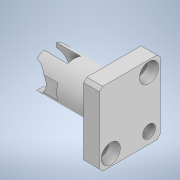
# Autodesk Inventor part: Фиксатор-11
Saved by Autodesk Inventor 2022 (Build 260153000, 153)
## iProperties
Created: 2021-12-02
Part Number: Фиксатор-11
Material: Типовые
Document SubType Name: Modeling
Designer: Украинцев
Density: 1 g/cm^3
Appearance: По умолчанию
Author: Украинцев
Autodesk Inventor part; units mm, degrees
ref_plane "YZ Plane" through (0, 0, 0) normal (1, 0, 0) x (0, 1, 0)
ref_plane "XZ Plane" through (0, 0, 0) normal (0, 1, 0) x (-1, 0, 0)
ref_plane "XY Plane" through (0, 0, 0) normal (0, 0, 1) x (1, 0, 0)
sketch "Эскиз1" plane through (0, 0, 0) normal (0, 1, 0) x (-1, 0, 0)
  line L0 (-5, -19) -> (5, -19)
  line L1 (5, -19) -> (5, 19)
  line L2 (5, 19) -> (-5, 19)
  line L3 (-5, 19) -> (-5, -19)
  line L4 (-5, -19) -> (5, 19) construction
  line L5 (5, -19) -> (-5, 19) construction
  line L6 (5, 0) -> (5, 12)
  line L7 (5, 12) -> (45, 12)
  line L8 (45, 12) -> (45, 0)
  line L9 (30, 0) -> (5, 0)
  line L10 (45, 0) -> (45, 4)
  line L11 (45, 4) -> (30, 4)
  line L12 (30, 4) -> (30, 0)
  line L13 (45, 12) -> (45, 11)
  line L14 (45, 11) -> (29, 11)
  line L15 (29, 11) -> (29, 12)
  line L16 (45, 4) -> (30, 4)
  line L17 (30, 4) -> (30, -4)
  line L18 (30, -4) -> (45, -4)
  line L19 (45, -4) -> (45, 4)
  line L20 (29, -11) -> (29, -12)
  line L21 (29, -12) -> (45, -12)
  line L22 (45, -12) -> (45, -11)
  line L23 (45, -11) -> (29, -11)
  line L24 (29, -11) -> (29, -12)
  line L25 (5, 12) -> (8, 12)
  line L26 (5, 0) -> (5, 11.75)
  line L27 (5, 11.75) -> (8, 11.75)
  line L28 (8, 11.75) -> (8, 12)
  line L29 (5, 11.75) -> (6, 11.75)
  line L30 (6, 11.75) -> (6, 12.75)
  line L31 (6, 12.75) -> (5, 12.75)
  line L32 (5, 12.75) -> (5, 11.75)
  circle A0 centre (6, 12.75) radius 1
  line L33 (8, 12) -> (6, 11.75)
  point P0 (0, 0)
  point P1 (6.2462, 11.7808)
  dimension "d0" = 10
  dimension "d1" = 38
  dimension "d2" = 12
  dimension "d3" = 40
  dimension "d4" = 4
  dimension "d5" = 15
  dimension "d6" = 1
  dimension "d7" = 16
  dimension "d13" = 8
  dimension "d14" = 22
  dimension "d15" = 1
  dimension "d60" = 3
  dimension "d61" = 11.75
  dimension "d62" = 1
  dimension "d63" = 1
  constraints: 68 end point, 12 perpendicular, 8 parallel, 6 point on line, 5 horizontal, 4 midpoint, 1 centre point, 1 coincident, 1 tangent
  measures "d0" distance of L2.end L1.end
  measures "d1" distance of L1.end L0.end
  measures "d2" distance of L6.start L6.end
  measures "d3" distance of L6.end L7.end
  measures "d4" distance of L8.end L10.end
  measures "d5" distance of L10.end L11.end
  measures "d6" distance of L7.end L13.end
  measures "d7" distance of L13.end L14.end
  measures "d13" distance of L17.end L16.end
  measures "d14" distance of L14.end L20.start
  measures "d15" distance of L20.start L20.end
  measures "d60" distance of L6.end L25.end
  measures "d61" distance of L6.start L26.end
  measures "d62" distance of L31.end L30.end
  measures "d63" distance of L30.end L29.end
extrude "Выдавливание1" add sketch "Эскиз1" along normal mid plane 46 contours L3 L2 L1 L0
revolve "Вращение1" add sketch "Эскиз1" angle 360 about axis through (-30, 0, 0) along (1, 0, 0) contours L1 L27 L28 L7 L15 L14 L8 L11 L12 L9 | L1 L7 A0 L27 | A0 L7 L1 | A0 L33 L28 L27 | L14 L15 L7 L8
extrude "Выдавливание3" cut sketch "Эскиз1" along normal mid plane 46 contours L12 L11 L8 L19 L18 L17 | L14 L15 L7 L8 | L23 L22 L21 L20
sketch "Эскиз3" plane through (-29, 4.7958, -11) normal (0, 0, -1) x (-1, 0, 0)
  line L0 (16, -9.5917) -> (16, 0) projected
  circle A0 centre (16, -4.7958) radius 8.5
  point P0 (-29, -4.7958)
  dimension "d21" = 17
  constraints: 1 centre point, 1 midpoint
  measures "d21" diameter of A0
extrude "Выдавливание5" cut sketch "Эскиз3" against normal blind 39
sketch "Эскиз4" plane through (5, -23, -19) normal (1, 0, 0) x (0, 0, -1)
  line L0 (-19, 23) -> (-19, 39)
  line L1 (-19, 39) -> (-31, 39)
  line L2 (-19, 23) -> (-19, 7)
  line L3 (-19, 7) -> (-7, 7)
  line L4 (-19, 7) -> (-31, 7)
  line L5 (-19, 39) -> (-7, 39)
  dimension "d24" = 16
  dimension "d25" = 12
  dimension "d26" = 16
  dimension "d27" = 12
  dimension "d28" = 12
  constraints: 12 end point, 4 coincident, 3 perpendicular, 2 vertical, 1 horizontal
  measures "d24" distance of L0.start L0.end
  measures "d25" distance of L0.end L1.end
  measures "d26" distance of L0.start L2.end
  measures "d27" distance of L2.end L3.end
  measures "d28" distance of L2.end L4.end
hole "Отверстие3" at (5, 16, -12) at (5, -16, 12) direction (-1, 0, 0) diameter 7 end through all counterbore diameter 12 counterbore depth 7
hole "Отверстие4" at (5, -16, -12) direction (-1, 0, 0) diameter 8 end through all
chamfer "Фаска1" distance 2 angle 45 4 edges at (0, 23, -19) (0, -23, -19) (0, -23, 19) (0, 23, 19)
